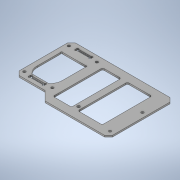
# Autodesk Inventor part: Trunk_upper_side_frame
Saved by Autodesk Inventor 2020.4 (Build 244396000, 396)
## iProperties
Created: 2022-01-02
Part Number: Trunk_upper_side_frame
Material: GFRP
Document SubType Name: Modeling
Designer: Masato Kubotera
Density: 1.75 g/cm^3
Appearance: 滑らか - 標準の灰色
Mass: 22.9321 g
Surface Area: 157.417 cm^2
Volume: 13.1041 cm^3
Description: GFRP T2
Author: Masato Kubotera
Autodesk Inventor part; units mm, degrees
ref_plane "YZ Plane" through (0, 0, 0) normal (1, 0, 0) x (0, 1, 0)
ref_plane "XZ Plane" through (0, 0, 0) normal (0, 1, 0) x (-1, 0, 0)
ref_plane "XY Plane" through (0, 0, 0) normal (0, 0, 1) x (1, 0, 0)
derived "Trunk_basis.ipt"
sketch "スケッチ1" plane through (0, 0, 0) normal (0, 1, 0) x (-1, 0, 0)
  line L0 (0, 22) -> (0, -142.9) construction
  circle A0 centre (5, 0) radius 10.5 construction
  line L1 (-7, 16) -> (36, 16) construction
  line L2 (36, 16) -> (36, -16) construction
  line L3 (36, -16) -> (-7, -16) construction
  line L4 (-7, -16) -> (-7, 16) construction
  line L5 (-7, 16) -> (36, -16) construction
  line L6 (36, 16) -> (-7, -16) construction
  line L7 (33, 13.5) -> (6, 13.5) construction
  line L8 (6, 13.5) -> (6, -13.5) construction
  line L9 (6, -13.5) -> (33, -13.5) construction
  line L10 (33, -13.5) -> (33, 13.5) construction
  line L11 (33, 13.5) -> (6, -13.5) construction
  line L12 (6, 13.5) -> (33, -13.5) construction
  line L13 (-7, 0) -> (36, 0) construction
  arc A1 (5, 16) -> (-7, 10.583) centre (5, 0) ccw construction
  line L14 (34.5651, -16.05) -> (5, -16.05) projected
  line L15 (5, 16.05) -> (34.5651, 16.05) projected
  line L16 (36.05, 14.5651) -> (36.05, -14.5651) projected
  line L17 (36.05, -16.05) -> (-7.05, 16.05) construction
  line L18 (-7.05, -16.05) -> (36.05, 16.05) construction
  arc A2 (5, 16.05) -> (-6.5314, 11.1638) centre (5, 0) ccw projected
  arc A3 (-6.5314, 11.1638) -> (-7.05, 9.8372) centre (-6.0721, 10.2196) ccw projected
  arc A4 (36.05, 14.5651) -> (34.5651, 16.05) centre (35.3075, 15.3075) ccw projected
  circle A5 centre (6, 13.5) radius 1.35 construction
  line L19 (19.5, 13.5) -> (19.5, -13.5) construction
  circle A6 centre (33, 13.5) radius 1.35 construction
  line L20 (-12, 22) -> (-17, 17) projected
  line L21 (-17, 17) -> (-17, -16) projected
  line L22 (-17, -16) -> (-28.5, -27.5) projected
  line L23 (-28.5, -27.5) -> (-28.5, -103) projected
  line L24 (54.5, -22.5) -> (54.5, 17) projected
  line L25 (54.5, 17) -> (49.5, 22) projected
  line L26 (49.5, 22) -> (-12, 22) projected
  line L27 (-35.5597, -116.5529) -> (-28.5, -142.9) projected
  line L28 (-16, -139) -> (-16, -94) construction
  line L29 (-7.5, -140.4849) -> (-7.5, -142.9) projected
  line L30 (-7.5, -142.9) -> (7.5, -142.9) projected
  line L31 (7.5, -140.4849) -> (7.5, -142.9) projected
  arc A7 (-7.5, -140.4849) -> (-8.9849, -139) centre (-8.2425, -139.7425) ccw projected
  line L32 (-17.5, -138.9955) -> (-17.5, -133) construction
  line L33 (-19, -133) -> (-16, -133) construction
  line L34 (-19, -133) -> (-19, -139) construction
  line L35 (-16, -133) -> (-16, -139) construction
  line L36 (-12, 22) -> (-7, 22) construction
  line L37 (-7, 22) -> (-7, -22) construction
  line L38 (-7, -22) -> (-12, -22) construction
  line L39 (-12, -22) -> (-12, 22) construction
  line L40 (-12, 22) -> (-7, -22) construction
  line L41 (-7, 22) -> (-12, -22) construction
  line L42 (-9.5, 22) -> (-9.5, -22) construction
  line L43 (-7, 0) -> (-12, 0) construction
  circle A8 centre (-9.5, 17.75) radius 1.6 projected
  line L44 (-12, 10) -> (-9.5, 10) construction
  line L45 (-9.5, 10) -> (-9.5, -10) construction
  line L46 (-9.5, -10) -> (-12, -10) construction
  line L47 (-12, -10) -> (-12, 10) construction
  line L48 (-12, 10) -> (-9.5, -10) construction
  line L49 (-9.5, 10) -> (-12, -10) construction
  line L50 (-9.45, 10.05) -> (-12.05, 10.05) projected
  line L51 (-12.05, 7.95) -> (-12.05, -7.95) projected
  line L52 (-12.05, -10.05) -> (-9.45, -10.05) projected
  line L53 (-9.45, -7.95) -> (-9.45, 7.95) projected
  line L54 (-9.45, 10.05) -> (-12.05, -10.05) construction
  line L55 (-12.05, 10.05) -> (-9.45, -10.05) construction
  arc A9 (-12.05, 10.05) -> (-12.05, 7.95) centre (-12.05, 9) ccw projected
  line L56 (-10.75, 10) -> (-10.75, -10) construction
  arc A10 (-9.45, 7.95) -> (-9.45, 10.05) centre (-9.45, 9) ccw projected
  circle A11 centre (-9.5, -17.75) radius 1.6 projected
  arc A12 (-12.05, -7.95) -> (-12.05, -10.05) centre (-12.05, -9) ccw projected
  arc A13 (-9.45, -10.05) -> (-9.45, -7.95) centre (-9.45, -9) ccw projected
  line L57 (36, 14.4) -> (44.5, 14.4) construction
  line L58 (44.5, 14.4) -> (44.5, -14.4) construction
  line L59 (36, -14.4) -> (44.5, -14.4) construction
  line L60 (46.95, 7.95) -> (46.95, -7.95) projected
  line L61 (49.5, 0) -> (44.5, 0) construction
  line L62 (44.5, 22) -> (49.5, 22) construction
  line L63 (49.55, -7.95) -> (49.55, 7.95) projected
  line L64 (48.25, 10) -> (48.25, -10) construction
  line L65 (49.5, 10) -> (47, -10) construction
  line L66 (49.5, -10) -> (47, -10) construction
  line L67 (49.5, 10) -> (49.5, -10) construction
  line L68 (47, 10) -> (49.5, -10) construction
  line L69 (46.95, -10.05) -> (49.55, -10.05) projected
  line L70 (46.95, 10.05) -> (49.55, -10.05) construction
  line L71 (49.55, 10.05) -> (46.95, -10.05) construction
  line L72 (49.5, -22) -> (44.5, -22) construction
  line L73 (44.5, 22) -> (49.5, -22) construction
  line L74 (49.5, 22) -> (49.5, -22) construction
  line L75 (49.5, 22) -> (44.5, -22) construction
  line L76 (47, 22) -> (47, -22) construction
  line L77 (44.5, -22) -> (44.5, 22) construction
  circle A14 centre (47, -17.75) radius 1.6 projected
  arc A15 (49.55, -10.05) -> (49.55, -7.95) centre (49.55, -9) ccw projected
  line L78 (47, -10) -> (47, 10) construction
  arc A16 (46.95, -7.95) -> (46.95, -10.05) centre (46.95, -9) ccw projected
  arc A17 (46.95, 10.05) -> (46.95, 7.95) centre (46.95, 9) ccw projected
  arc A18 (49.55, 7.95) -> (49.55, 10.05) centre (49.55, 9) ccw projected
  line L79 (47, 10) -> (49.5, 10) construction
  line L80 (49.55, 10.05) -> (46.95, 10.05) projected
  circle A19 centre (47, 17.75) radius 1.6 projected
  circle A20 centre (5, 0) radius 16 construction
  arc A21 (-6.5314, -11.1638) -> (5, -16.05) centre (5, 0) ccw projected
  arc A22 (-7.05, -9.8372) -> (-6.5314, -11.1638) centre (-6.0721, -10.2196) ccw projected
  arc A23 (34.5651, -16.05) -> (36.05, -14.5651) centre (35.3075, -15.3075) ccw projected
  line L81 (-7.05, -9.8372) -> (-7.05, 9.8372) projected
  line L82 (17.5, -138.9955) -> (17.5, -133) construction
  line L83 (19, -133) -> (19, -139) construction
  line L84 (16, -133) -> (16, -139) construction
  line L85 (19, -133) -> (16, -133) construction
  circle A24 centre (6, -13.5) radius 1.35 projected
  circle A25 centre (33, -13.5) radius 1.35 projected
  line L86 (-25.5, -142.9) -> (-7.5, -142.9) construction
  line L87 (25.5, -142.9) -> (7.5, -142.9) construction
  line L88 (-23.5, -22.5) -> (54.5, -22.5) construction
  line L89 (54.5, -22.5) -> (54.5, -103) projected
  circle A26 centre (-13.5, -55) radius 1.75 projected
  line L90 (-16.5, -59) -> (42.5, -59) projected
  line L91 (44.5, -61) -> (44.5, -88) projected
  line L92 (42.5, -90) -> (-16.5, -90) projected
  line L93 (-18.5, -88) -> (-18.5, -61) projected
  line L94 (-18.5, -59) -> (44.5, -90) construction
  line L95 (44.5, -59) -> (-18.5, -90) construction
  line L96 (-16.5, -27.5) -> (42.5, -27.5) projected
  line L97 (44.5, -29.5) -> (44.5, -49) projected
  line L98 (42.5, -51) -> (-16.5, -51) projected
  line L99 (-18.5, -49) -> (-18.5, -29.5) projected
  line L100 (-18.5, -27.5) -> (44.5, -51) construction
  line L101 (44.5, -27.5) -> (-18.5, -51) construction
  line L102 (-23.5, -108) -> (-28.5, -103) projected
  circle A27 centre (-20.5415, -102) radius 1.6 projected
  line L103 (-25.7227, -96) -> (25.7227, -96) projected
  line L104 (25.7227, -96) -> (34.9603, -112) projected
  line L105 (35.5597, -116.5529) -> (28.5, -142.9) projected
  line L106 (-25.7227, -96) -> (-34.9603, -112) projected
  line L107 (54.5, -103) -> (49.5, -108) projected
  arc A28 (-16.5, -27.5) -> (-18.5, -29.5) centre (-16.5, -29.5) ccw projected
  arc A29 (-18.5, -49) -> (-16.5, -51) centre (-16.5, -49) ccw projected
  arc A30 (42.5, -51) -> (44.5, -49) centre (42.5, -49) ccw projected
  arc A31 (44.5, -29.5) -> (42.5, -27.5) centre (42.5, -29.5) ccw projected
  arc A32 (-16.5, -59) -> (-18.5, -61) centre (-16.5, -61) ccw projected
  arc A33 (-18.5, -88) -> (-16.5, -90) centre (-16.5, -88) ccw projected
  arc A34 (42.5, -90) -> (44.5, -88) centre (42.5, -88) ccw projected
  arc A35 (44.5, -61) -> (42.5, -59) centre (42.5, -61) ccw projected
  line L108 (-23.5, -108) -> (49.5, -108) projected
  line L109 (-25.5, -139) -> (-25.5, -142.9) projected
  line L110 (-25.5, -142.9) -> (-28.5, -142.9) projected
  line L111 (-17.9813, -99.3843) -> (-16.9961, -101.0907) projected
  line L112 (-16.9961, -102.9093) -> (-17.9813, -104.6157) projected
  line L113 (-19.5563, -105.525) -> (-21.5266, -105.525) projected
  line L114 (-23.1016, -104.6157) -> (-24.0868, -102.9093) projected
  line L115 (-24.0868, -101.0907) -> (-23.1016, -99.3843) projected
  line L116 (-21.5266, -98.475) -> (-19.5563, -98.475) projected
  line L117 (-16, -94) -> (16, -94) construction
  arc A36 (-24.0868, -101.0907) -> (-24.0868, -102.9093) centre (-23.5618, -102) ccw projected
  arc A37 (-23.1016, -104.6157) -> (-21.5266, -105.525) centre (-22.0516, -104.6157) ccw projected
  arc A38 (-19.5563, -105.525) -> (-17.9813, -104.6157) centre (-19.0313, -104.6157) ccw projected
  arc A39 (-16.9961, -102.9093) -> (-16.9961, -101.0907) centre (-17.5211, -102) ccw projected
  arc A40 (-17.9813, -99.3843) -> (-19.5563, -98.475) centre (-19.0313, -99.3843) ccw projected
  arc A41 (-21.5266, -98.475) -> (-23.1016, -99.3843) centre (-22.0516, -99.3843) ccw projected
  line L118 (16, -139) -> (16, -94) construction
  line L119 (16, -94) -> (-16, -94) construction
  line L120 (-25.5, -139) -> (-8.9849, -139) projected
  line L121 (25.5, -142.9) -> (28.5, -142.9) projected
  arc A42 (8.9849, -139) -> (7.5, -140.4849) centre (8.2425, -139.7425) ccw projected
  circle A43 centre (29.7641, -115) radius 1.25 projected
  line L122 (33.4891, -124.2803) -> (21.898, -121.1745) projected
  line L123 (29.7641, -115) -> (25.623, -130.4548) projected
  circle A44 centre (29.7641, -115) radius 6 projected
  circle A45 centre (-20.5415, -102) radius 6 construction
  line L124 (1.9319, -109.4824) -> (7.5588, -130.4824) projected
  line L125 (5.6269, -133) -> (-5.6269, -133) projected
  line L126 (5.3151, -110.5176) -> (10.942, -131.5176) projected
  line L127 (12.8739, -133) -> (17.1947, -133) projected
  line L128 (19.1266, -131.5176) -> (24.7535, -110.5176) projected
  line L129 (22.8217, -108) -> (7.2469, -108) projected
  circle A46 centre (25.623, -130.4548) radius 1.25 projected
  circle A47 centre (25.623, -130.4548) radius 6 construction
  line L130 (-1.9319, -109.4824) -> (-7.5588, -130.4824) projected
  arc A48 (1.9319, -109.4824) -> (-1.9319, -109.4824) centre (0, -110) ccw projected
  arc A49 (-7.5588, -130.4824) -> (-5.6269, -133) centre (-5.6269, -131) ccw projected
  arc A50 (5.6269, -133) -> (7.5588, -130.4824) centre (5.6269, -131) ccw projected
  arc A51 (7.2469, -108) -> (5.3151, -110.5176) centre (7.2469, -110) ccw projected
  arc A52 (24.7535, -110.5176) -> (22.8217, -108) centre (22.8217, -110) ccw projected
  arc A53 (17.1947, -133) -> (19.1266, -131.5176) centre (17.1947, -131) ccw projected
  arc A54 (10.942, -131.5176) -> (12.8739, -133) centre (12.8739, -131) ccw projected
  arc A55 (-5.3151, -110.5176) -> (-7.2469, -108) centre (-7.2469, -110) ccw projected
  line L131 (-22.8217, -108) -> (-7.2469, -108) projected
  line L132 (-5.3151, -110.5176) -> (-10.942, -131.5176) projected
  arc A56 (-22.8217, -108) -> (-24.7535, -110.5176) centre (-22.8217, -110) ccw projected
  line L133 (-19.1266, -131.5176) -> (-24.7535, -110.5176) projected
  arc A57 (-19.1266, -131.5176) -> (-17.1947, -133) centre (-17.1947, -131) ccw projected
  line L134 (-12.8739, -133) -> (-17.1947, -133) projected
  arc A58 (-12.8739, -133) -> (-10.942, -131.5176) centre (-12.8739, -131) ccw projected
  circle A59 centre (-29.7641, -115) radius 1.25 projected
  circle A60 centre (-25.623, -130.4548) radius 1.25 projected
  arc A61 (35.5597, -116.5529) -> (34.9603, -112) centre (29.7641, -115) ccw projected
  arc A62 (-34.9603, -112) -> (-35.5597, -116.5529) centre (-29.7641, -115) ccw projected
  arc A63 (-24.0151, -139) -> (-25.5, -140.4849) centre (-24.7575, -139.7425) ccw projected
  line L135 (25.5, -139) -> (25.5, -142.9) projected
  arc A64 (25.5, -140.4849) -> (24.0151, -139) centre (24.7575, -139.7425) ccw projected
  line L136 (25.5, -139) -> (8.9849, -139) projected
  line L137 (21.5266, -98.475) -> (19.5563, -98.475) projected
  line L138 (16.9961, -102.9093) -> (17.9813, -104.6157) projected
  arc A65 (21.5266, -105.525) -> (23.1016, -104.6157) centre (22.0516, -104.6157) ccw projected
  circle A66 centre (20.5415, -102) radius 1.6 projected
  line L139 (24.0868, -101.0907) -> (23.1016, -99.3843) projected
  arc A67 (24.0868, -102.9093) -> (24.0868, -101.0907) centre (23.5618, -102) ccw projected
  line L140 (23.1016, -104.6157) -> (24.0868, -102.9093) projected
  arc A68 (23.1016, -99.3843) -> (21.5266, -98.475) centre (22.0516, -99.3843) ccw projected
  line L141 (19.5563, -105.525) -> (21.5266, -105.525) projected
  arc A69 (19.5563, -98.475) -> (17.9813, -99.3843) centre (19.0313, -99.3843) ccw projected
  arc A70 (17.9813, -104.6157) -> (19.5563, -105.525) centre (19.0313, -104.6157) ccw projected
  line L142 (17.9813, -99.3843) -> (16.9961, -101.0907) projected
  arc A71 (16.9961, -101.0907) -> (16.9961, -102.9093) centre (17.5211, -102) ccw projected
  line L143 (16, -139) -> (16, -94) construction
  circle A72 centre (20.5415, -102) radius 6 construction
  arc A73 (29.5045, -117.5445) -> (31.2612, -117.0738) centre (30.247, -116.802) ccw construction
  line L144 (31.8379, -116.4971) -> (31.2612, -117.0738) construction
  line L145 (29.5045, -117.5445) -> (28.7167, -117.3334) construction
  arc A74 (27.4307, -116.0474) -> (28.7167, -117.3334) centre (28.4449, -116.3192) ccw construction
  line L146 (27.4307, -116.0474) -> (27.2196, -115.2596) construction
  line L147 (27.6903, -113.5029) -> (28.267, -112.9262) construction
  arc A75 (30.0237, -112.4555) -> (28.267, -112.9262) centre (29.2813, -113.198) ccw construction
  arc A76 (27.6903, -113.5029) -> (27.2196, -115.2596) centre (27.9621, -114.5171) ccw construction
  line L148 (30.0237, -112.4555) -> (30.8116, -112.6666) construction
  arc A77 (31.8379, -116.4971) -> (32.3086, -114.7404) centre (31.5662, -115.4829) ccw construction
  arc A78 (32.0975, -113.9526) -> (30.8116, -112.6666) centre (31.0833, -113.6808) ccw construction
  line L149 (32.0975, -113.9526) -> (32.3086, -114.7404) construction
  point P0 (0, 0)
  point P1 (14.5, 0)
  point P2 (19.5, 0)
  point P3 (-7.05, 10.6019)
  point P4 (19.5, 0)
  point P5 (-9.5, 0)
  point P6 (-10.75, 0)
  point P7 (36.05, 14.4)
  point P8 (36.05, -14.4)
  point P9 (48.25, 0)
  point P10 (47, 0)
  point P11 (13, -74.5)
  point P12 (13, -39.25)
  point P13 (15.5276, -102)
  point P14 (15.5276, -139)
  point P15 (-18.5063, -98.475)
  point P16 (-16.4711, -102)
  point P17 (-18.5063, -105.525)
  point P18 (-22.5766, -105.525)
  point P19 (-22.5766, -98.475)
  point P20 (-24.6118, -102)
  point P21 (-22.5766, -105.525)
  point P22 (-18.5063, -105.525)
  point P23 (-16.4711, -102)
  point P24 (-18.5063, -98.475)
  point P25 (-22.5766, -98.475)
  point P26 (27.6936, -122.7274)
  point P27 (0, -102.2726)
  point P28 (0, -133)
  point P29 (-7.5, -139)
  point P30 (-22.5766, -98.475)
  point P31 (18.5063, -98.475)
  point P32 (18.5063, -98.475)
  point P33 (22.5766, -105.525)
  point P34 (22.5766, -105.525)
  point P35 (24.6118, -102)
  point P36 (22.5766, -98.475)
  point P37 (22.5766, -98.475)
  point P38 (22.5766, -98.475)
  point P39 (18.5063, -105.525)
  point P40 (16.4711, -102)
  point P41 (16.4711, -102)
  point P42 (18.5063, -105.525)
  point P43 (29.7641, -115)
  point P44 (29.7641, -115)
  point P45 (30.5187, -117.8163)
  point P46 (30.5187, -117.8163)
  point P47 (27.7025, -117.0617)
  point P48 (27.7025, -117.0617)
  point P49 (31.8258, -112.9383)
  point P50 (26.9479, -114.2454)
  point P51 (29.0095, -112.1837)
  point P52 (29.0095, -112.1837)
  point P53 (31.8258, -112.9383)
  point P54 (29.0095, -112.1837)
  point P55 (32.5804, -115.7546)
  constraints: 4 other
extrude "押し出し1" add sketch "スケッチ1" along normal blind 2 contours L26 L25 L24 L89 L107 L108 L104 L103 L106 L23 L22 L21 L20 | L106 L103 L104 L108 L102 L23 | L111 A39 L112 A38 L113 A37 L114 A36 L115 A41 L116 A40 | A68 L139 A67 L140 A65 L141 A70 L138 A71 L142 A69 L137
